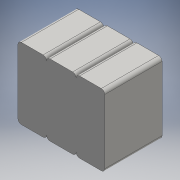
# Autodesk Inventor part: Simplistic_battery_pack_batteryspace-spencermical
Saved by Autodesk Inventor 2016 (Build 200138000, 138)
## iProperties
Created: 2016-03-10
Part Number: Simplistic_battery_pack_batteryspace-spencermical
Material: Generic
Document SubType Name: Modeling
Designer: Spencer
Density: 1 g/cm^3
Appearance: Default
Author: Spencer
Autodesk Inventor part; units mm, degrees
ref_plane "YZ Plane" through (0, 0, 0) normal (1, 0, 0) x (0, 1, 0)
ref_plane "XZ Plane" through (0, 0, 0) normal (0, 1, 0) x (-1, 0, 0)
ref_plane "XY Plane" through (0, 0, 0) normal (0, 0, 1) x (1, 0, 0)
sketch "Sketch1" plane through (0, 0, 0) normal (0, 1, 0) x (-1, 0, 0)
  line L0 (0, 0) -> (-50, 0)
  line L1 (-50, 0) -> (-50, -35)
  line L2 (-50, -35) -> (0, -35)
  line L3 (0, -35) -> (0, 0)
  dimension "d0" = 35
  dimension "d1" = 50
  constraints: 8 end point, 2 parallel, 1 horizontal, 1 perpendicular
  measures "d0" distance of L2.end L0.start
  measures "d1" distance of L0.start L0.end
extrude "Extrusion1" add sketch "Sketch1" along normal blind 33
sketch "Sketch2" plane through (0, 0, 0) normal (0, 0, 1) x (1, 0, 0)
  line L0 (0, 33) -> (50, 33) projected
  line L1 (16.5, 33) -> (16.5, 0)
  line L2 (0, 0) -> (50, 0) projected
  line L3 (33.5, 33) -> (33.5, 0)
  line L4 (0, 0) -> (0, 33) projected
  line L5 (50, 0) -> (50, 33) projected
  line L6 (0, 0) -> (0, 33) projected
  line L7 (0, 33) -> (16.5, 33)
  line L8 (16.5, 33) -> (16.5, 0)
  line L9 (16.5, 0) -> (0, 0)
  line L10 (0, 0) -> (0, 33)
  line L11 (33.5, 33) -> (50, 33)
  line L12 (50, 33) -> (50, 0)
  line L13 (50, 0) -> (33.5, 0)
  line L14 (33.5, 0) -> (33.5, 33)
  dimension "d4" = 16.5
  dimension "d5" = 16.5
  constraints: 20 end point, 5 parallel, 4 point on line, 2 horizontal, 2 perpendicular, 1 vertical
  measures "d4" distance from line of L1.start L4
  measures "d5" distance from line of L3.start L5
extrude "Extrusion2" add sketch "Sketch2" along normal blind 3 contours L0 L1 L2 L4 | L0 L5 L2 L3
fillet "Fillet1" radius 2 4 edges at (0, 16.5, 3) (16.5, 16.5, 3) (33.5, 16.5, 3) (50, 16.5, 3)
sketch "Sketch3" plane through (16.5, 0, 0) normal (0, 0, 1) x (1, 0, 0)
  line L0 (0, 33) -> (17, 33) projected
  line L1 (17, 0) -> (17, 33) projected
  line L2 (0, 33) -> (17, 33)
  line L3 (17, 33) -> (17, 0)
  line L4 (17, 0) -> (0, 0)
  line L5 (0, 0) -> (0, 33)
  point P0 (-16.5, 0)
  constraints: 8 end point, 2 parallel, 1 horizontal, 1 perpendicular
extrude "Extrusion3" add sketch "Sketch3" along normal blind 3
fillet "Fillet2" radius 2 2 edges at (16.5, 16.5, 3) (33.5, 16.5, 3)
sketch "Sketch4" plane through (50, 0, -35) normal (0, 0, -1) x (-1, 0, 0)
  line L0 (0, 0) -> (50, 0) projected
  line L1 (33.5, 0) -> (33.5, 33)
  line L2 (0, 33) -> (50, 33) projected
  line L3 (14.5, 0) -> (2, 0) projected
  line L4 (16.5, 0) -> (16.5, 33)
  line L5 (50, 0) -> (50, 33) projected
  line L6 (0, 0) -> (0, 33) projected
  line L7 (50, 0) -> (33.5, 0)
  line L8 (33.5, 0) -> (33.5, 33)
  line L9 (33.5, 33) -> (50, 33)
  line L10 (50, 33) -> (50, 0)
  line L11 (16.5, 0) -> (14.5, 0) projected
  line L12 (16.5, 0) -> (0, 0)
  line L13 (0, 0) -> (0, 33)
  line L14 (0, 33) -> (16.5, 33)
  line L15 (16.5, 33) -> (16.5, 0)
  dimension "d12" = 16.5
  dimension "d13" = 16.5
  constraints: 20 end point, 5 parallel, 4 point on line, 2 horizontal, 2 perpendicular, 1 vertical
  measures "d12" distance from line of L1.start L5
  measures "d13" distance from line of L4.start L6
extrude "Extrusion4" add sketch "Sketch4" along normal blind 3 contours L6 L2 L4 L0 | L2 L5 L0 L1
fillet "Fillet3" radius 2 4 edges at (0, 16.5, -38) (16.5, 16.5, -38) (33.5, 16.5, -38) (50, 16.5, -38)
sketch "Sketch5" plane through (33.5, 0, -35) normal (0, 0, -1) x (-1, 0, 0)
  line L0 (17, 0) -> (17, 33) projected
  line L1 (-2, 33) -> (0, 33) projected
  line L2 (17, 0) -> (0, 0)
  line L3 (0, 0) -> (0, 33)
  line L4 (0, 33) -> (17, 33)
  line L5 (17, 33) -> (17, 0)
  point P0 (33.5, 0)
  constraints: 8 end point, 2 parallel, 1 horizontal, 1 perpendicular
extrude "Extrusion5" add sketch "Sketch5" along normal blind 3
fillet "Fillet4" radius 2 2 edges at (16.5, 16.5, -38) (33.5, 16.5, -38)
body "Solid1"
